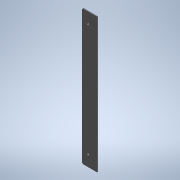
# Autodesk Inventor part: Deckelanschlag
Saved by Autodesk Inventor 2021.3 (Build 253353000, 353)
## iProperties
Created: 2021-10-19
Part Number: Deckelanschlag
Material: Generisch
Document SubType Name: Modeling
Designer: bhelg
Density: 1 g/cm^3
Appearance: Vorgabe
Author: bhelg
Autodesk Inventor part; units mm, degrees
ref_plane "YZ Plane" through (0, 0, 0) normal (1, 0, 0) x (0, 1, 0)
ref_plane "XZ Plane" through (0, 0, 0) normal (0, 1, 0) x (-1, 0, 0)
ref_plane "XY Plane" through (0, 0, 0) normal (0, 0, 1) x (1, 0, 0)
sketch "Skizze1" plane through (0, 0, 0) normal (0, 1, 0) x (-1, 0, 0)
  line L0 (0, 0) -> (40, 0)
  line L1 (40, 0) -> (40, -1.5)
  line L2 (40, -1.5) -> (0, -1.5)
  line L3 (0, -1.5) -> (0, 0)
  dimension "d0" = 40
  dimension "d1" = 1.5
  constraints: 8 end point, 2 parallel, 1 horizontal, 1 perpendicular
  measures "d0" distance of L1.end L2.end
  measures "d1" distance of L0.end L1.end
extrude "Extrusion1" add sketch "Skizze1" along normal blind 298
sketch "Skizze2" plane through (-40, 0, 0) normal (0, 0, 1) x (1, 0, 0)
  line L0 (0, 298) -> (40, 298) projected
  line L1 (40, 0) -> (40, 298) projected
  point P0 (20, 24)
  point P1 (20, 274)
  dimension "d4" = 250
  dimension "d5" = 298
  dimension "d6" = 24
  dimension "d7" = 20
  dimension "d8" = 20
  measures "d4" distance of point (20, 274) point (20, 24)
  measures "d5" distance from line of L0 L1.start
  measures "d6" distance from line of L0 point (20, 274)
  measures "d7" distance from line of point (20, 274) L1
  measures "d8" distance from line of L1 point (20, 24)
hole "Bohrung1" at (-20, 24, 0) at (-20, 274, 0) direction (0, 0, -1) diameter 4.5 depth 11.8 tip angle 118
sketch "Skizze3" plane through (-40, 0, 0) normal (0, 0, 1) x (1, 0, 0)
  line L0 (0, 0) -> (0, 298) projected
  line L1 (0, 0) -> (7, 0)
  line L2 (7, 0) -> (7, 298)
  line L3 (7, 298) -> (0, 298)
  line L4 (0, 298) -> (0, 0)
  point P0 (40, 0)
  dimension "d16" = 7
  dimension "d17" = 298
  constraints: 8 end point, 2 parallel, 1 horizontal, 1 perpendicular
  measures "d16" distance of L3.end L2.end
  measures "d17" distance of L2.end L1.end
extrude "Extrusion2" cut sketch "Skizze3" against normal blind 298
fillet "Rundung1" radius 3 2 edges at (-33, 0, -0.75) (-33, 298, -0.75)
